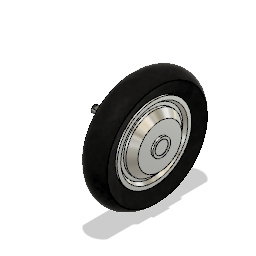
01part (Autodesk Fusion 360 design; units mm, degrees)
Autodesk Fusion 360 part; units mm, degrees
sketch "Sketch1" plane through (0, 0, 0) normal (0, 0, 1) x (1, 0, 0)
  line L0 (-5, 14) -> (-5, 22)
  line L1 (-5, 22) -> (4, 22)
  line L2 (4, 22) -> (4, 45)
  line L3 (4, 45) -> (21, 62)
  line L4 (21, 62) -> (21, 72)
  line L5 (21, 72) -> (15, 72)
  line L6 (15, 72) -> (15, 80)
  line L7 (15, 80) -> (19, 80)
  line L8 (19, 80) -> (19, 76)
  line L9 (19, 76) -> (51, 76)
  line L10 (51, 76) -> (51, 80)
  line L11 (51, 80) -> (55, 80)
  line L12 (55, 80) -> (55, 72)
  line L13 (55, 72) -> (49, 67)
  line L14 (49, 67) -> (49, 60)
  line L15 (49, 60) -> (54, 60)
  line L16 (54, 60) -> (67, 47)
  line L17 (67, 47) -> (67, 19)
  line L18 (67, 19) -> (71, 19)
  line L19 (71, 19) -> (71, 14)
  line L20 (71, 14) -> (70.4, 14)
  line L21 (70.4, 14) -> (70.4, 0)
  line L22 (70.4, 0) -> (0, 0)
  line L23 (0, 0) -> (0, 14)
  line L24 (0, 14) -> (-5, 14)
  dimension "d1" = 14
  dimension "d2" = 8
  dimension "d3" = 9
  dimension "d4" = 23
  dimension "d5" = 17
  dimension "d6" = 17
  dimension "d7" = 10
  dimension "d8" = 6
  dimension "d9" = 4
  dimension "d10" = 8
  dimension "d12" = 7
  dimension "d13" = 6
  dimension "d14" = 5
  dimension "d15" = 5
  dimension "d16" = 13
  dimension "d17" = 13
  dimension "d18" = 28
  dimension "d19" = 4
  dimension "d20" = 5
  dimension "d21" = 0.6
  dimension "d22" = 40
  dimension "d39" = 5
  constraint vertical L0
  constraint perpendicular L0 L1
  constraint perpendicular L1 L2
  constraint perpendicular L1 L4
  constraint perpendicular L4 L5
  constraint perpendicular L5 L6
  constraint perpendicular L4 L7
  constraint perpendicular L7 L8
  constraint perpendicular L8 L9
  constraint perpendicular L9 L10
  constraint perpendicular L8 L11
  constraint perpendicular L11 L14
  constraint perpendicular L14 L15
  constraint perpendicular L15 L17
  constraint parallel L15 L18
  constraint perpendicular L18 L19
  constraint perpendicular L19 L20
  constraint perpendicular L20 L21
  constraint perpendicular L21 L22
  constraint perpendicular L22 L23
  constraint perpendicular L0 L24
  constraint vertical L12
  constraint equal L6 L12
  constraint equal L7 L11
  constraint collinear L7 L11
  constraint equal L7 L8
  constraint coincident L22.end L23.start
  measures "d1" distance of L22.end L23.end
  measures "d2" distance of L0.start L0.end
  measures "d3" distance of L0.end L1.end
  measures "d4" distance of L1.end L2.end
  measures "d5" vertical distance of L2.end L3.end
  measures "d6" horizontal distance of L2.end L3.end
  measures "d7" distance of L3.end L4.end
  measures "d8" distance of L4.end L5.end
  measures "d9" distance of L6.end L7.end
  measures "d10" distance of L5.end L6.end
  measures "d12" distance of L13.end L14.end
  measures "d13" horizontal distance of L12.end L13.end
  measures "d14" vertical distance of L12.end L13.end
  measures "d15" distance of L14.end L15.end
  measures "d16" horizontal distance of L15.end L16.end
  measures "d17" vertical distance of L15.end L16.end
  measures "d18" distance of L16.end L17.end
  measures "d19" distance of L17.end L18.end
  measures "d20" distance of L18.end L19.end
  measures "d21" distance of L19.end L20.end
  measures "d22" distance of L6 L12
  measures "d39" distance of L0.start L23.end
revolve "Revolve1" add sketch "Sketch1" angle 360 about axis through (1.75, 0, 0) along (1, 0, 0) makes body 1
sketch "Sketch2" plane through (0, 0, 0) normal (0, 0, 1) x (1, 0, 0)
  line L0 (51, 80) -> (61.5, 108)
  line L1 (-1.394, 122) -> (67.606, 122) construction
  line L2 (51, 80) -> (55, 80) construction
  line L3 (35, 129) -> (35, 53) construction
  line L4 (15, 72) -> (15, 80) construction
  line L5 (55, 80) -> (55, 72) construction
  line L6 (51, 80) -> (51, 76)
  line L7 (51, 76) -> (19, 76)
  line L8 (19, 76) -> (19, 80)
  line L9 (19, 80) -> (8.5, 108)
  arc A0 (61.5, 108) -> (8.5, 108) centre (35, 89.9196) ccw
  point P0 (51, 76)
  point P1 (19, 76)
  point P2 (19, 80)
  dimension "d29" = 42
  dimension "d30" = 28
  dimension "d31" = 53
  constraint horizontal L1
  constraint tangent L1 A0
  constraint perpendicular L1 L3
  constraint symmetric L3 L4 L5
  constraint coincident A0.centre L3
  constraint coincident L0.start L2.start
  constraint coincident P0 L6.end
  constraint coincident P1 L7.end
  constraint coincident P2 L8.end
  constraint equal L0 L9
  measures "d29" distance of L1 L2
  measures "d30" vertical distance of L0.end L0.start
  measures "d31" distance of L0.end L9.end
revolve "Revolve2" add sketch "Sketch2" angle 360 about axis through (1.75, 0, 0) along (1, 0, 0) separate body makes body 2
sketch "Sketch3" plane through (0, 0, 0) normal (0, 0, 1) x (1, 0, 0)
  line L0 (35.2097, 3) -> (-74, 3)
  line L1 (-74, 3) -> (-74, 8)
  line L2 (-74, 8) -> (-22, 8)
  line L3 (-22, 8) -> (-22, 8.3)
  line L4 (-22, 8.3) -> (35.2097, 8.3)
  line L5 (35.2097, 8.3) -> (35.2097, 3)
  line L6 (70.4, 0) -> (0, 0)
  line L7 (-74, 0) -> (12.1646, 0) construction
  line L8 (-5, 14) -> (-5, 22) construction
  dimension "d33" = 52
  dimension "d34" = 8
  dimension "d35" = 8.3
  dimension "d36" = 5
  dimension "d37" = 69
  constraint perpendicular L0 L1
  constraint perpendicular L1 L2
  constraint perpendicular L0 L3
  constraint perpendicular L1 L4
  constraint horizontal L0
  constraint perpendicular L0 L5
  constraint coincident L6 L7.end
  measures "d33" distance of L1.end L2.end
  measures "d34" distance of L2 L7
  measures "d35" distance of L4 L7
  measures "d36" distance of L0.end L1.end
  measures "d37" distance of L1 L8
revolve "Revolve3" add sketch "Sketch3" angle 360 about axis through (1.75, 0, 0) along (1, 0, 0) separate body makes body 3
ref_plane "WorkPlane1" through (-61.2975, 0, 8) normal (0, 0, 1) x (0, 1, 0)
sketch "Sketch4" plane through (0, 0, 0) normal (0, 0, 1) x (1, 0, 0)
  line L0 (-72.2, 8) -> (-27.2, 8)
  line L1 (-27.2, 8) -> (-27.2, 5)
  line L2 (-27.2, 5) -> (-72.2, 5)
  line L3 (-72.2, 5) -> (-72.2, 8)
  line L4 (-74, -8) -> (-74, 8)
  line L5 (-74, 8) -> (-22, 8)
  dimension "d41" = 45
  dimension "d42" = 1.8
  dimension "d43" = 3
  constraint horizontal L0
  constraint vertical L1
  constraint horizontal L2
  constraint vertical L3
  constraint coincident L0.start L5
  measures "d41" distance of L0.start L0.end
  measures "d42" distance of L3 L4
  measures "d43" distance of L0.start L2.end
extrude "Extrude1" cut sketch "Sketch4" along normal mid plane 20 bodies 3
chamfer "Chamfer1" distance 1 angle 45 1 edges at (-74, -2.8929, 7.4586) on bodies 3
named bodies: "диск", "покрышка", "ось"
